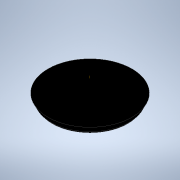
# Autodesk Inventor part: Microphone_iGOKU
Saved by Autodesk Inventor 2021.3 (Build 253353000, 353)
## iProperties
Created: 2021-05-26
Part Number: Microphone_iGOKU
Material: 一般
Document SubType Name: Modeling
Designer: gisen
Density: 1 g/cm^3
Appearance: 陽極酸化 - 黒
Author: gisen
Autodesk Inventor part; units mm, degrees
ref_plane "YZ Plane" through (0, 0, 0) normal (1, 0, 0) x (0, 1, 0)
ref_plane "XZ Plane" through (0, 0, 0) normal (0, 1, 0) x (-1, 0, 0)
ref_plane "XY Plane" through (0, 0, 0) normal (0, 0, 1) x (1, 0, 0)
sketch "スケッチ3" plane through (0, 0, 0) normal (0, 0, 1) x (1, 0, 0)
  line L0 (0, 0) -> (0, 16.5989)
  line L1 (-26.75, 0) -> (26.75, 0)
  line L2 (0, 0) -> (-26.75, 0)
  line L3 (-26.75, 0) -> (-26.75, 1.32)
  line L4 (29.75, 1.32) -> (-29.75, 1.32)
  line L5 (-27.77, 1.32) -> (-29.75, 5.4388)
  line L6 (-29.75, 1.32) -> (-29.75, 14.6)
  line L7 (-29.75, 14.6) -> (0, 14.6)
  arc A0 (0, 14.6) -> (-29.75, 5.4388) centre (1.1553, -42.0372) ccw
  line L8 (0, -53.7814) -> (0, 28.4277)
  dimension "d7" = 53.5
  dimension "d8" = 59.5
  dimension "d10" = 4.57
  dimension "d11" = 14.6
  constraints: 18 end point, 4 point on line, 2 perpendicular, 2 point on circle, 1 centre point, 1 collinear, 1 vertical
  measures "d7" distance of L1.start L1.end
  measures "d8" distance of L4.start L4.end
  measures "d10" distance of L5.start L5.end
  measures "d11" distance from line of L6.end L1
revolve "回転1" add sketch "スケッチ3" angle 360 about axis through (0, -53.7814, 0) along (0, 1, 0) contours L1 L3 L4 L0 | L4 L5 A0 L0
